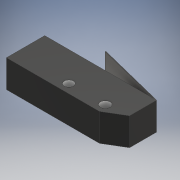
# Autodesk Inventor part: microswitch
Saved by Autodesk Inventor 2018.3 (Build 223284000, 284)
## iProperties
Created: 2019-01-01
Part Number: microswitch
Material: ABS プラスチック
Document SubType Name: Modeling
Designer: shun2
Density: 1.06 g/cm^3
Appearance: 滑らか - 白
Author: shun2
Autodesk Inventor part; units mm, degrees
ref_plane "YZ Plane" through (0, 0, 0) normal (1, 0, 0) x (0, 1, 0)
ref_plane "XZ Plane" through (0, 0, 0) normal (0, 1, 0) x (-1, 0, 0)
ref_plane "XY Plane" through (0, 0, 0) normal (0, 0, 1) x (1, 0, 0)
sketch "スケッチ1" plane through (0, 0, 0) normal (0, 0, 1) x (1, 0, 0)
  line L0 (0, 0) -> (24.2856, 0)
  line L1 (29.2, 2.9323) -> (29.2, 10)
  line L2 (28.3778, 10) -> (0, 10)
  line L3 (0, 10) -> (0, 0)
  circle A0 centre (23.5, 2.3) radius 1.25
  circle A1 centre (14, 2.3) radius 1.175
  line L4 (29.2, 2.9323) -> (24.2856, 0)
  line L5 (29.2, 10) -> (11.5467, 14.4273)
  line L6 (11.5467, 14.4273) -> (11.4981, 14.2333)
  line L7 (11.4981, 14.2333) -> (28.3778, 10)
  dimension "d2" = 2.5
  dimension "d3" = 2.35
  dimension "d4" = 18.2
  dimension "d5" = 0.2
  constraints: 16 end point, 3 perpendicular, 2 centre point, 2 parallel, 1 coincident, 1 horizontal
  measures "d2" diameter of A0
  measures "d3" diameter of A1
  measures "d4" distance of L1.end L5.end
  measures "d5" distance of L5.end L6.end
extrude "押し出し1" add sketch "スケッチ1" along normal blind 7.2
